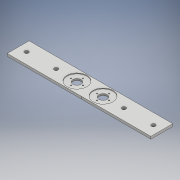
# Autodesk Inventor part: Drivetrainsideinside
Saved by Autodesk Inventor 2017 (Build 210142000, 142)
## iProperties
Created: 2016-10-15
Part Number: Drivetrainsideinside
Material: Generic
Document SubType Name: Modeling
Designer: Kevin G
Density: 1 g/cm^3
Appearance: Default
Author: Kevin G
Autodesk Inventor part; units mm, degrees
ref_plane "YZ Plane" through (0, 0, 0) normal (1, 0, 0) x (0, 1, 0)
ref_plane "XZ Plane" through (0, 0, 0) normal (0, 1, 0) x (-1, 0, 0)
ref_plane "XY Plane" through (0, 0, 0) normal (0, 0, 1) x (1, 0, 0)
sketch "Sketch1" plane through (0, 0, 0) normal (0, 0, 1) x (1, 0, 0)
  line L0 (-275.4313, -42) -> (-275.4313, 42)
  circle A0 centre (-243.408, 0) radius 7.5
  circle A1 centre (-130.124, 0) radius 7.5
  circle A2 centre (-50.0124, 0) radius 15.875
  circle A3 centre (-50.0124, 23.0188) radius 2.3813
  circle A4 centre (-26.9936, 0) radius 2.3813
  circle A5 centre (-73.0311, 0) radius 2.3813
  circle A6 centre (-50.0124, -23.0187) radius 2.3813
  line L1 (-275.4313, 42) -> (9.5034, 42)
  line L2 (-275.4313, -42) -> (9.5252, -42)
  line L3 (275.4312, -41.9309) -> (275.4312, 42.0691)
  line L4 (275.4312, 42.0691) -> (9.5034, 42)
  line L5 (275.4312, -41.9309) -> (9.5252, -42)
  circle A7 centre (-50.0124, 0) radius 38.1
  circle A8 centre (243.4084, 0) radius 7.5
  circle A9 centre (130.1244, 0) radius 7.5
  circle A10 centre (50.0128, 0) radius 15.875
  circle A11 centre (50.0123, 23.0188) radius 2.3813
  circle A12 centre (26.9936, 0) radius 2.3813
  circle A13 centre (73.0311, 0) radius 2.3813
  circle A14 centre (50.0123, -23.0187) radius 2.3813
  circle A15 centre (50.0128, 0) radius 38.1
  dimension "d4" = 15
  dimension "d7" = 15
  dimension "d9" = 31.75
  dimension "d11" = 4.7625
  dimension "d13" = 4.7625
  dimension "d15" = 23.0188
  dimension "d16" = 4.7625
  dimension "d18" = 4.7625
  dimension "d25" = 550.8625
  dimension "d50" = 23.0188
  dimension "d51" = 23.0188
  dimension "d52" = 23.0188
  dimension "d53" = 80.1116
  dimension "d54" = 113.284
  dimension "d62" = 76.2
  dimension "d88" = 84
  dimension "d89" = 42
  dimension "d90" = 42
  dimension "d91" = 32.0233
  dimension "d92" = 42
  dimension "d93" = 42
  dimension "d97" = 100.0252
  dimension "d98" = 80.1116
  dimension "d99" = 113.284
  dimension "d100" = 32.0228
  constraints: 16 centre point, 12 end point, 2 coincident, 1 horizontal
  measures "d4" diameter of A0
  measures "d7" diameter of A1
  measures "d9" diameter of A2
  measures "d11" diameter of A3
  measures "d13" diameter of A4
  measures "d15" distance of A2.centre A5.centre
  measures "d16" diameter of A5
  measures "d18" diameter of A6
  measures "d25" distance between parallel lines of L0 L3
  measures "d50" distance of A3.centre A2.centre
  measures "d51" distance of A4.centre A2.centre
  measures "d52" distance of A2.centre A6.centre
  measures "d53" distance of A2.centre A1.centre
  measures "d54" distance of A0.centre A1.centre
  measures "d62" diameter of A7
  measures "d88" distance between parallel lines of L5 L4
  measures "d89" distance from line of L1 A2.centre
  measures "d90" distance from line of L2 A7.centre
  measures "d91" distance from line of L0 A0.centre
  measures "d92" distance from line of L1 A0.centre
  measures "d93" distance from line of L2 A1.centre
  measures "d97" distance of A15.centre A7.centre
  measures "d98" distance of A9.centre A10.centre
  measures "d99" distance of A8.centre A9.centre
  measures "d100" distance from line of L3 A8.centre
extrude "Extrusion4" add sketch "Sketch1" along normal blind 9.525 contours L0 L1 L4 L3 L5 L2 | A7 | A15
sketch "Sketch5" plane through (0, 0, 9.525) normal (0, 0, 1) x (1, 0, 0)
  line L0 (-275.4313, -42) -> (-275.4313, 42)
  circle A0 centre (-243.408, 0) radius 7.5
  circle A1 centre (-130.124, 0) radius 7.5
  circle A2 centre (-50.0124, 0) radius 15.875
  circle A3 centre (-50.0124, 23.0188) radius 2.3813
  circle A4 centre (-26.9936, 0) radius 2.3813
  circle A5 centre (-73.0311, 0) radius 2.3813
  circle A6 centre (-50.0124, -23.0187) radius 2.3813
  line L1 (-275.4313, 42) -> (9.5034, 42)
  line L2 (-275.4313, -42) -> (9.5143, -42)
  line L3 (275.4312, -41.9309) -> (9.5143, -42)
  line L4 (275.4312, 42.0691) -> (9.5034, 42)
  line L5 (275.4312, -41.9309) -> (275.4312, 42.0691)
  circle A7 centre (-50.0124, 0) radius 38.1
  circle A8 centre (50.0123, -23.0187) radius 2.3813
  circle A9 centre (50.0123, 23.0188) radius 2.3813
  circle A10 centre (26.9936, 0) radius 2.3813
  circle A11 centre (50.0128, 0) radius 15.875
  circle A12 centre (73.0311, 0) radius 2.3813
  circle A13 centre (50.0128, 0) radius 38.1
  circle A14 centre (130.1244, 0) radius 7.5
  circle A15 centre (243.4084, 0) radius 7.5
  point P0 (0, 0)
  dimension "d103" = 15
  dimension "d104" = 15
  dimension "d105" = 31.75
  dimension "d106" = 4.7625
  dimension "d107" = 4.7625
  dimension "d108" = 23.0188
  dimension "d109" = 4.7625
  dimension "d110" = 4.7625
  dimension "d111" = 550.8625
  dimension "d112" = 23.0188
  dimension "d113" = 23.0188
  dimension "d114" = 23.0188
  dimension "d115" = 80.1116
  dimension "d116" = 113.284
  dimension "d117" = 76.2
  dimension "d118" = 84
  dimension "d119" = 42
  dimension "d120" = 42
  dimension "d121" = 32.0233
  dimension "d122" = 42
  dimension "d123" = 42
  dimension "d124" = 100.0252
  dimension "d125" = 80.1116
  dimension "d126" = 113.284
  dimension "d127" = 32.0228
  constraints: 16 centre point, 12 end point, 2 coincident, 1 horizontal
  measures "d103" diameter of A0
  measures "d104" diameter of A1
  measures "d105" diameter of A2
  measures "d106" diameter of A3
  measures "d107" diameter of A4
  measures "d108" distance of A2.centre A5.centre
  measures "d109" diameter of A5
  measures "d110" diameter of A6
  measures "d111" distance between parallel lines of L0 L5
  measures "d112" distance of A3.centre A2.centre
  measures "d113" distance of A4.centre A2.centre
  measures "d114" distance of A2.centre A6.centre
  measures "d115" distance of A2.centre A1.centre
  measures "d116" distance of A0.centre A1.centre
  measures "d117" diameter of A7
  measures "d118" distance between parallel lines of L3 L4
  measures "d119" distance from line of L1 A2.centre
  measures "d120" distance from line of L2 A7.centre
  measures "d121" distance from line of L0 A0.centre
  measures "d122" distance from line of L1 A0.centre
  measures "d123" distance from line of L2 A1.centre
  measures "d124" distance of A13.centre A7.centre
  measures "d125" distance of A14.centre A11.centre
  measures "d126" distance of A15.centre A14.centre
  measures "d127" distance from line of L5 A15.centre
emboss "Emboss4" sketch "Sketch5" operation cut depth 3 direction (0, 0, -1) contours A7 | A13
body "Solid4"
